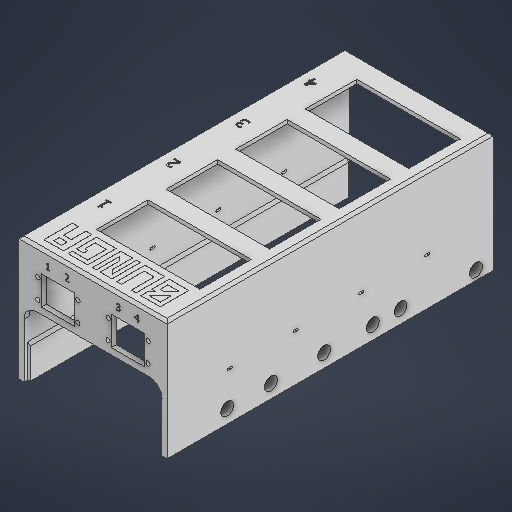
# Autodesk Inventor part: QuadSupply
Saved by Autodesk Inventor 2026 (Build 300175050, 175E)
## iProperties
Created: 2025-08-17
Part Number: QuadSupply
Material: Generic
Document SubType Name: Modeling
Designer: user
Density: 1 g/cm^3
Appearance: Default
Author: user
## iProperties of the stored document QuadSupply_3DPrint.ipt
Created: 2025-08-17
Part Number: QuadSupply_3DPrint
Material: Generic
Document SubType Name: Modeling
Designer: user
Density: 1 g/cm^3
Appearance: Default
Author: user
Autodesk Inventor part; units mm, degrees
ref_plane "YZ Plane" through (0, 0, 0) normal (1, 0, 0) x (0, 1, 0)
ref_plane "XZ Plane" through (0, 0, 0) normal (0, 1, 0) x (-1, 0, 0)
ref_plane "XY Plane" through (0, 0, 0) normal (0, 0, 1) x (1, 0, 0)
sketch "Sketch1" plane through (0, 0, 0) normal (0, 1, 0) x (-1, 0, 0)
  line L0 (54.5, -128.75) -> (-54.5, -128.75) construction
  line L1 (-54.5, -128.75) -> (-54.5, 128.75) construction
  line L2 (-54.5, 128.75) -> (54.5, 128.75) construction
  line L3 (54.5, 128.75) -> (54.5, -128.75) construction
  line L4 (58.5, -128.75) -> (-58.5, -128.75)
  line L5 (-58.5, -128.75) -> (-58.5, 128.75)
  line L6 (-58.5, 128.75) -> (58.5, 128.75)
  line L7 (58.5, 128.75) -> (58.5, -128.75)
  line L8 (32.1, -111.75) -> (-49.5, -111.75)
  line L9 (-49.5, -111.75) -> (-49.5, -71.15)
  line L10 (-49.5, -71.15) -> (32.1, -71.15)
  line L11 (32.1, -71.15) -> (32.1, -111.75)
  point P0 (0, 0)
  point P1 (-54.5, 0)
  point P2 (0, -128.75)
  point P3 (0, -128.75)
  point P4 (-58.5, 0)
  dimension "d0" = 109
  dimension "d1" = 257.5
  dimension "d3" = 4
  dimension "d4" = 40.6
  dimension "d5" = 81.6
  dimension "d6" = 17
  dimension "d56" = 5
  constraints: 24 end point, 6 parallel, 4 midpoint, 3 horizontal, 3 perpendicular, 2 horizontal alignment, 2 vertical alignment, 1 collinear
  measures "d0" distance of L0.start L0.end
  measures "d1" distance of L2.end L0.start
  measures "d3" distance between parallel lines of L3 L7
  measures "d4" distance of L10.end L8.start
  measures "d5" distance of L8.start L8.end
  measures "d6" distance between parallel lines of L4 L8
  measures "d56" distance between parallel lines of L1 L9
extrude "Extrusion1" add sketch "Sketch1" against normal blind 3 contours L4 L5 L6 L7 | L8 L9 L10 L11
extrude "Extrusion2" cut sketch "Sketch1" against normal up to surface (3 mm away) contours L8 L9 L10 L11
pattern_linear "Rectangular Pattern1" count 4 spacing 55 along (0, 0, 1) of "Extrusion2"
sketch "Sketch2" plane through (0, -3, 0) normal (0, -1, 0) x (1, 0, 0)
  line L0 (-58.5, -128.75) -> (-58.5, 128.75) projected
  line L1 (58.5, -128.75) -> (-58.5, -128.75) projected
  line L2 (-58.5, 128.75) -> (-54.5, 128.75)
  line L3 (-54.5, 128.75) -> (-54.5, -128.75)
  line L4 (-54.5, -128.75) -> (-58.5, -128.75)
  line L5 (-58.5, -128.75) -> (-58.5, 128.75)
  point P0 (0, 0)
  dimension "d15" = 4
  constraints: 8 end point, 2 parallel, 1 horizontal, 1 perpendicular, 1 point on line
  measures "d15" distance between parallel lines of L0 L3
extrude "Extrusion3" add sketch "Sketch2" along normal blind 95
sketch "Sketch3" plane through (-54.5, -3, 128.75) normal (1, 0, 0) x (0, 0, -1)
  line L0 (3, -69) -> (254.5, -69)
  line L1 (254.5, -69) -> (254.5, -95)
  line L2 (254.5, -95) -> (3, -95)
  line L3 (3, -95) -> (3, -69)
  line L4 (257.5, -95) -> (0, -95) projected
  point P0 (128.75, 3)
  point P1 (128.75, -95)
  dimension "d18" = 251.5
  dimension "d19" = 26
  constraints: 8 end point, 2 midpoint, 2 parallel, 1 horizontal, 1 perpendicular
  measures "d18" distance of L0.start L0.end
  measures "d19" distance between parallel lines of L2 L0
extrude "Extrusion4" add sketch "Sketch3" along normal blind 2
sketch "Sketch5" plane through (0, -3, 0) normal (0, -1, 0) x (1, 0, 0)
  line L0 (54.5, 128.75) -> (58.5, 128.75)
  line L1 (58.5, 128.75) -> (58.5, -128.75)
  line L2 (58.5, -128.75) -> (54.5, -128.75)
  line L3 (54.5, -128.75) -> (54.5, 128.75)
  point P0 (0, 0)
  dimension "d24" = 4
  constraints: 8 end point, 2 coincident, 2 parallel, 1 horizontal, 1 perpendicular
  measures "d24" distance between parallel lines of L1 L3
extrude "Extrusion5" add sketch "Sketch5" along normal blind 91.1
sketch "Sketch6" plane through (54.5, -3, -128.75) normal (-1, 0, 0) x (0, 0, 1)
  line L0 (3, -72.8) -> (254.5, -72.8)
  line L1 (254.5, -72.8) -> (254.5, -91.1)
  line L2 (254.5, -91.1) -> (3, -91.1)
  line L3 (3, -91.1) -> (3, -72.8)
  line L4 (257.5, -91.1) -> (0, -91.1) projected
  point P0 (128.75, 3)
  point P1 (128.75, -91.1)
  dimension "d27" = 251.5
  dimension "d28" = 18.3
  constraints: 8 end point, 2 midpoint, 2 parallel, 1 horizontal, 1 perpendicular
  measures "d27" distance of L0.start L0.end
  measures "d28" distance between parallel lines of L0 L2
extrude "Extrusion6" add sketch "Sketch6" along normal blind 3
sketch "Sketch7" plane through (51.5, -3, -128.75) normal (-1, 0, 0) x (0, 0, 1)
  line L0 (3, -72.8) -> (3, -91.1) projected
  line L1 (3, -91.1) -> (254.5, -91.1) projected
  line L2 (254.5, -91.1) -> (254.5, -72.8) projected
  line L3 (254.5, -72.8) -> (3, -72.8) projected
  line L4 (3, -80.6) -> (254.5, -80.6) construction
  line L5 (257.5, 0) -> (257.5, -91.1) projected
  circle A0 centre (210, -80.6) radius 5
  circle A1 centre (175.5, -80.6) radius 5
  circle A2 centre (133.5, -80.6) radius 5
  circle A3 centre (95, -80.6) radius 5
  circle A4 centre (73, -80.6) radius 5
  circle A5 centre (13.5, -83.9) radius 5
  point P0 (128.75, 3)
  dimension "d31" = 10.5
  dimension "d34" = 47.5
  dimension "d35" = 82
  dimension "d37" = 124
  dimension "d39" = 162.5
  dimension "d41" = 184.5
  dimension "d42" = 10
  dimension "d43" = 244
  dimension "d44" = 7.2
  constraints: 7 point on line, 6 centre point, 5 equal radius, 2 end point, 1 horizontal
  measures "d31" distance between parallel lines of L1 L4
  measures "d34" distance from line of L5 A0.centre
  measures "d35" distance from line of L5 A1.centre
  measures "d37" distance from line of L5 A2.centre
  measures "d39" distance from line of L5 A3.centre
  measures "d41" distance from line of L5 A4.centre
  measures "d42" diameter of A5
  measures "d43" distance from line of L5 A5.centre
  measures "d44" distance from line of L1 A5.centre
extrude "Extrusion7" cut sketch "Sketch7" against normal up to surface (7 mm away) contours A0 | A1 | A2 | A3 | A4 | A5
sketch "Sketch8" plane through (-58.5, 0, -128.75) normal (-1, 0, 0) x (0, 0, 1)
  line L0 (0, -58) -> (257.5, -58) construction
  line L1 (0, 0) -> (0, -98) projected
  line L2 (257.5, 0) -> (257.5, -98) projected
  line L3 (257.5, -98) -> (0, -98) projected
  line L4 (50.85, -57.15) -> (53.15, -57.15) construction
  line L5 (50.85, -58) -> (53.15, -58)
  line L6 (53.15, -56.3) -> (50.85, -56.3)
  arc A0 (50.85, -56.3) -> (50.85, -58) centre (50.85, -57.15) ccw
  arc A1 (53.15, -58) -> (53.15, -56.3) centre (53.15, -57.15) ccw
  point P0 (128.75, 0)
  point P1 (52, -57.15)
  point P2 (54, -57.15)
  point P3 (50, -57.15)
  point P4 (52, -58)
  dimension "d47" = 40
  dimension "d48" = 1.7
  dimension "d49" = 4
  dimension "d50" = 52
  constraints: 10 end point, 6 point on circle, 4 tangent, 3 point on line, 2 centre point, 2 horizontal, 2 midpoint, 1 parallel
  measures "d47" distance between parallel lines of L3 L0
  measures "d48" distance between parallel lines of L5 L6
  measures "d49" distance of point (54, -57.15) point (50, -57.15)
  measures "d50" distance from line of L1 point (52, -57.15)
extrude "Extrusion8" cut sketch "Sketch8" against normal up to surface (117 mm away)
pattern_linear "Rectangular Pattern2" count 4 spacing 52 along (0, 0, 1) of "Extrusion8"
sketch "Sketch9" plane through (-58.5, 0, 128.75) normal (0, 0, 1) x (1, 0, 0)
  line L0 (0, 0) -> (117, 0) projected
  line L1 (0, 0) -> (0, -98) projected
  line L2 (117, 0) -> (0, 0)
  line L3 (0, 0) -> (0, -45)
  line L4 (0, -45) -> (117, -45)
  line L5 (117, -45) -> (117, 0)
  point P0 (58.5, 0)
  dimension "d57" = 45
  constraints: 8 end point, 2 parallel, 1 horizontal, 1 perpendicular, 1 point on line
  measures "d57" distance between parallel lines of L0 L4
extrude "Extrusion9" add sketch "Sketch9" against normal blind 4
sketch "Sketch10" plane through (-58.5, 0, 128.75) normal (0, 0, 1) x (1, 0, 0)
  line L0 (15, -20.85) -> (46.6, -20.85) construction
  line L1 (46.6, -20.85) -> (46.6, -36.35) construction
  line L2 (46.6, -36.35) -> (15, -36.35) construction
  line L3 (15, -36.35) -> (15, -20.85) construction
  circle A0 centre (15, -20.85) radius 1.65
  circle A1 centre (46.6, -20.85) radius 1.65
  circle A2 centre (15, -36.35) radius 1.65
  circle A3 centre (46.6, -36.35) radius 1.65
  line L4 (17.6, -17.2) -> (44, -17.2)
  line L5 (44, -17.2) -> (44, -40)
  line L6 (44, -40) -> (17.6, -40)
  line L7 (17.6, -40) -> (17.6, -17.2)
  line L8 (4, -45) -> (113, -45) projected
  line L9 (0, 0) -> (0, -98) projected
  line L10 (70.4, -20.85) -> (102, -20.85) construction
  line L11 (102, -20.85) -> (102, -36.35) construction
  line L12 (102, -36.35) -> (70.4, -36.35) construction
  line L13 (70.4, -36.35) -> (70.4, -20.85) construction
  circle A4 centre (70.4, -20.85) radius 1.65
  circle A5 centre (102, -20.85) radius 1.65
  circle A6 centre (70.4, -36.35) radius 1.65
  circle A7 centre (102, -36.35) radius 1.65
  line L14 (73, -17.2) -> (99.4, -17.2)
  line L15 (99.4, -17.2) -> (99.4, -40)
  line L16 (99.4, -40) -> (73, -40)
  line L17 (73, -40) -> (73, -17.2)
  line L18 (117, 0) -> (117, -94.1) projected
  point P0 (58.5, 0)
  point P1 (30.8, -20.85)
  point P2 (30.8, -17.2)
  point P3 (44, -28.6)
  point P4 (46.6, -28.6)
  point P5 (86.2, -20.85)
  point P6 (86.2, -17.2)
  point P7 (99.4, -28.6)
  point P8 (102, -28.6)
  dimension "d60" = 31.6
  dimension "d61" = 15.5
  dimension "d62" = 3.3
  dimension "d63" = 26.4
  dimension "d64" = 22.8
  dimension "d65" = 5
  dimension "d66" = 15
  dimension "d67" = 31.6
  dimension "d68" = 15.5
  dimension "d69" = 3.3
  dimension "d70" = 26.4
  dimension "d71" = 22.8
  dimension "d72" = 15
  dimension "d73" = 5
  constraints: 32 end point, 8 centre point, 8 coincident, 8 midpoint, 8 parallel, 6 equal radius, 4 horizontal, 4 perpendicular, 2 horizontal alignment, 2 vertical alignment
  measures "d60" distance of L0.start L0.end
  measures "d61" distance of L2.end L0.start
  measures "d62" diameter of A0
  measures "d63" distance of L4.start L4.end
  measures "d64" distance of L4.end L5.end
  measures "d65" distance between parallel lines of L8 L6
  measures "d66" distance between parallel lines of L9 L3
  measures "d67" distance of L13.end L11.start
  measures "d68" distance of L13.start L13.end
  measures "d69" diameter of A4
  measures "d70" distance of L14.start L14.end
  measures "d71" distance of L14.end L15.end
  measures "d72" distance between parallel lines of L18 L11
  measures "d73" distance between parallel lines of L8 L16
extrude "Extrusion10" cut sketch "Sketch10" against normal up to surface (4 mm away)
sketch "Sketch11" plane through (-58.5, 0, 128.75) normal (0, 0, 1) x (1, 0, 0)
  line L0 (20.9646, -7.3633) -> (24.7195, -7.3633) construction
  line L1 (24.7195, -7.3633) -> (24.7195, -12.4045) construction
  line L2 (24.7195, -12.4045) -> (20.9646, -12.4045) construction
  line L3 (20.9646, -12.4045) -> (20.9646, -7.3633) construction
  line L4 (36.1808, -7.3633) -> (39.9357, -7.3633) construction
  line L5 (39.9357, -7.3633) -> (39.9357, -12.4045) construction
  line L6 (39.9357, -12.4045) -> (36.1808, -12.4045) construction
  line L7 (36.1808, -12.4045) -> (36.1808, -7.3633) construction
  line L8 (76.6169, -7.3633) -> (80.3717, -7.3633) construction
  line L9 (80.3717, -7.3633) -> (80.3717, -12.4045) construction
  line L10 (80.3717, -12.4045) -> (76.6169, -12.4045) construction
  line L11 (76.6169, -12.4045) -> (76.6169, -7.3633) construction
  line L12 (91.1541, -7.3633) -> (94.9089, -7.3633) construction
  line L13 (94.9089, -7.3633) -> (94.9089, -12.4045) construction
  line L14 (94.9089, -12.4045) -> (91.1541, -12.4045) construction
  line L15 (91.1541, -12.4045) -> (91.1541, -7.3633) construction
  line L16 (24.164, -12.3833) -> (21.7229, -12.3833)
  line L17 (21.7229, -12.3833) -> (21.7229, -11.8724)
  line L18 (21.7229, -11.8724) -> (22.6312, -11.8724)
  line L19 (22.6312, -11.8724) -> (22.6312, -8.519)
  line L20 (22.6312, -8.519) -> (21.7229, -8.519)
  line L21 (21.7229, -8.519) -> (21.7229, -8.0608)
  spline S0 degree 2 poles (21.7229, -8.0608) (22.2379, -8.0608) (22.7245, -7.7688) (22.7569, -7.3633) knots 0 0 0 1 2 2 2
  line L22 (22.7569, -7.3633) -> (23.2759, -7.3633)
  line L23 (23.2759, -7.3633) -> (23.2759, -11.8724)
  line L24 (23.2759, -11.8724) -> (24.164, -11.8724)
  line L25 (24.164, -11.8724) -> (24.164, -12.3833)
  line L26 (39.6315, -12.4725) -> (36.5457, -12.4725)
  line L27 (36.5457, -12.4725) -> (36.5457, -11.7629)
  spline S1 degree 2 poles (36.5457, -11.7629) (36.8782, -11.4507) (37.4703, -10.8708) (37.7541, -10.5586) knots 0 0 0 1 2 2 2
  spline S2 degree 2 poles (37.7541, -10.5586) (38.3258, -9.9301) (38.7435, -9.1759) (38.7435, -8.7744) knots 0 0 0 1 2 2 2
  spline S3 degree 2 poles (38.7435, -8.7744) (38.7435, -8.5636) (38.6137, -8.2473) (38.4962, -8.1459) knots 0 0 0 1 2 2 2
  spline S4 degree 2 poles (38.4962, -8.1459) (38.3786, -8.0445) (38.0704, -7.9432) (37.8839, -7.9432) knots 0 0 0 1 2 2 2
  spline S5 degree 2 poles (37.8839, -7.9432) (37.7054, -7.9432) (37.3405, -8.0324) (37.1742, -8.1013) knots 0 0 0 1 2 2 2
  spline S6 degree 2 poles (37.1742, -8.1013) (37.0323, -8.1581) (36.7688, -8.3203) (36.6877, -8.377) knots 0 0 0 1 2 2 2
  line L28 (36.6877, -8.377) -> (36.6512, -8.377)
  line L29 (36.6512, -8.377) -> (36.6512, -7.6634)
  spline S7 degree 2 poles (36.6512, -7.6634) (36.858, -7.562) (37.6, -7.3633) (37.9325, -7.3633) knots 0 0 0 1 2 2 2
  spline S8 degree 2 poles (37.9325, -7.3633) (38.634, -7.3633) (39.4247, -8.1054) (39.4247, -8.7379) knots 0 0 0 1 2 2 2
  spline S9 degree 2 poles (39.4247, -8.7379) (39.4247, -9.0339) (39.2869, -9.5286) (39.1652, -9.7395) knots 0 0 0 1 2 2 2
  spline S10 degree 2 poles (39.1652, -9.7395) (39.0436, -9.9585) (38.6908, -10.3883) (38.4962, -10.5951) knots 0 0 0 1 2 2 2
  spline S11 degree 2 poles (38.4962, -10.5951) (38.1799, -10.9398) (37.4054, -11.6778) (37.1742, -11.8927) knots 0 0 0 1 2 2 2
  line L30 (37.1742, -11.8927) -> (39.6315, -11.8927)
  line L31 (39.6315, -11.8927) -> (39.6315, -12.4725)
  spline S12 degree 2 poles (78.3321, -7.9432) (78.1496, -7.9432) (77.7887, -8.0324) (77.6144, -8.1013) knots 0 0 0 1 2 2 2
  spline S13 degree 2 poles (77.6144, -8.1013) (77.4522, -8.1702) (77.2129, -8.3162) (77.1197, -8.3811) knots 0 0 0 1 2 2 2
  line L32 (77.1197, -8.3811) -> (77.0791, -8.3811)
  line L33 (77.0791, -8.3811) -> (77.0791, -7.6715)
  spline S14 degree 2 poles (77.0791, -7.6715) (77.2981, -7.5539) (78.0483, -7.3633) (78.3848, -7.3633) knots 0 0 0 1 2 2 2
  spline S15 degree 2 poles (78.3848, -7.3633) (78.7254, -7.3633) (79.2323, -7.5012) (79.4391, -7.6472) knots 0 0 0 1 2 2 2
  spline S16 degree 2 poles (79.4391, -7.6472) (79.6581, -7.8053) (79.8852, -8.2635) (79.8852, -8.5717) knots 0 0 0 1 2 2 2
  spline S17 degree 2 poles (79.8852, -8.5717) (79.8852, -8.9853) (79.3418, -9.6097) (78.9606, -9.6908) knots 0 0 0 1 2 2 2
  line L34 (78.9606, -9.6908) -> (78.9606, -9.7395)
  spline S18 degree 2 poles (78.9606, -9.7395) (79.1188, -9.7719) (79.4797, -9.9179) (79.6337, -10.0639) knots 0 0 0 1 2 2 2
  spline S19 degree 2 poles (79.6337, -10.0639) (79.7878, -10.2058) (79.9825, -10.66) (79.9825, -10.9884) knots 0 0 0 1 2 2 2
  spline S20 degree 2 poles (79.9825, -10.9884) (79.9825, -11.325) (79.7513, -11.8967) (79.5405, -12.1157) knots 0 0 0 1 2 2 2
  spline S21 degree 2 poles (79.5405, -12.1157) (79.3215, -12.3428) (78.7011, -12.578) (78.3078, -12.578) knots 0 0 0 1 2 2 2
  spline S22 degree 2 poles (78.3078, -12.578) (77.9307, -12.578) (77.1927, -12.3955) (76.9413, -12.2698) knots 0 0 0 1 2 2 2
  line L35 (76.9413, -12.2698) -> (76.9413, -11.5602)
  line L36 (76.9413, -11.5602) -> (76.9899, -11.5602)
  spline S23 degree 2 poles (76.9899, -11.5602) (77.2008, -11.7143) (77.9145, -11.9981) (78.2672, -11.9981) knots 0 0 0 1 2 2 2
  spline S24 degree 2 poles (78.2672, -11.9981) (78.474, -11.9981) (78.8876, -11.8683) (79.0255, -11.7183) knots 0 0 0 1 2 2 2
  spline S25 degree 2 poles (79.0255, -11.7183) (79.1593, -11.5683) (79.3012, -11.2114) (79.3012, -10.9398) knots 0 0 0 1 2 2 2
  spline S26 degree 2 poles (79.3012, -10.9398) (79.3012, -10.6681) (79.1431, -10.3153) (79.0012, -10.2139) knots 0 0 0 1 2 2 2
  spline S27 degree 2 poles (79.0012, -10.2139) (78.8593, -10.1126) (78.474, -10.0355) (78.247, -10.0355) knots 0 0 0 1 2 2 2
  line L37 (78.247, -10.0355) -> (77.9631, -10.0355)
  line L38 (77.9631, -10.0355) -> (77.9631, -9.48)
  line L39 (77.9631, -9.48) -> (78.1861, -9.48)
  spline S28 degree 2 poles (78.1861, -9.48) (78.6362, -9.48) (79.2039, -9.0502) (79.2039, -8.6406) knots 0 0 0 1 2 2 2
  spline S29 degree 2 poles (79.2039, -8.6406) (79.2039, -8.45) (79.0579, -8.1783) (78.9404, -8.0972) knots 0 0 0 1 2 2 2
  spline S30 degree 2 poles (78.9404, -8.0972) (78.8146, -8.0121) (78.5065, -7.9432) (78.3321, -7.9432) knots 0 0 0 1 2 2 2
  line L40 (94.7386, -10.6478) -> (94.1425, -10.6478)
  line L41 (94.1425, -10.6478) -> (94.1425, -12.3671)
  line L42 (94.1425, -12.3671) -> (93.4978, -12.3671)
  line L43 (93.4978, -12.3671) -> (93.4978, -10.6478)
  line L44 (93.4978, -10.6478) -> (91.2879, -10.6478)
  line L45 (91.2879, -10.6478) -> (91.2879, -9.9422)
  line L46 (91.2879, -9.9422) -> (93.5262, -7.3633)
  line L47 (93.5262, -7.3633) -> (94.1425, -7.3633)
  line L48 (94.1425, -7.3633) -> (94.1425, -10.1085)
  line L49 (94.1425, -10.1085) -> (94.7386, -10.1085)
  line L50 (94.7386, -10.1085) -> (94.7386, -10.6478)
  line L51 (93.4978, -10.1085) -> (93.4978, -8.154)
  line L52 (93.4978, -8.154) -> (91.815, -10.1085)
  line L53 (91.815, -10.1085) -> (93.4978, -10.1085)
  point P0 (58.5, 0)
  point P1 (24.7195, -9.8839)
  point P2 (36.1808, -9.8839)
  point P3 (76.6169, -9.8839)
  point P4 (91.1541, -9.8839)
  dimension "d0" = 109
  dimension "d1" = 257.5
  dimension "d3" = 4
  dimension "d4" = 40.6
  dimension "d5" = 81.6
  dimension "d6" = 17
  dimension "d56" = 5
  constraints: 4 midpoint, 3 collinear, 3 horizontal alignment, 8 other
extrude "Extrusion11" cut sketch "Sketch11" against normal blind 0.5
sketch "Sketch12" plane through (0, 0, 0) normal (0, 1, 0) x (1, 0, 0)
  line L0 (-43.6132, -77.5449) -> (-49.3868, -77.5449) construction
  line L1 (-49.3868, -77.5449) -> (-49.3868, -69.5551) construction
  line L2 (-49.3868, -69.5551) -> (-43.6132, -69.5551) construction
  line L3 (-43.6132, -69.5551) -> (-43.6132, -77.5449) construction
  line L4 (-44.2509, -22.5844) -> (-48.7491, -22.5844) construction
  line L5 (-48.7491, -22.5844) -> (-48.7491, -14.5156) construction
  line L6 (-48.7491, -14.5156) -> (-44.2509, -14.5156) construction
  line L7 (-44.2509, -14.5156) -> (-44.2509, -22.5844) construction
  line L8 (-44.2764, 32.2784) -> (-48.7236, 32.2784) construction
  line L9 (-48.7236, 32.2784) -> (-48.7236, 40.6216) construction
  line L10 (-48.7236, 40.6216) -> (-44.2764, 40.6216) construction
  line L11 (-44.2764, 40.6216) -> (-44.2764, 32.2784) construction
  line L12 (-44.7542, 87.4582) -> (-48.2458, 87.4582) construction
  line L13 (-48.2458, 87.4582) -> (-48.2458, 95.4418) construction
  line L14 (-48.2458, 95.4418) -> (-44.7542, 95.4418) construction
  line L15 (-44.7542, 95.4418) -> (-44.7542, 87.4582) construction
  line L16 (-32.1, -93.85) -> (-32.1, -53.25) projected
  line L17 (-32.1, -38.85) -> (-32.1, 1.75) projected
  line L18 (-32.1, 16.15) -> (-32.1, 56.75) projected
  line L19 (-32.1, 71.15) -> (-32.1, 111.75) projected
  line L20 (-58.5, 128.75) -> (-58.5, -128.75) projected
  line L21 (-48.7289, -69.5179) -> (-44.8257, -69.5179)
  line L22 (-44.8257, -69.5179) -> (-44.8257, -70.3349)
  line L23 (-44.8257, -70.3349) -> (-46.278, -70.3349)
  line L24 (-46.278, -70.3349) -> (-46.278, -75.697)
  line L25 (-46.278, -75.697) -> (-44.8257, -75.697)
  line L26 (-44.8257, -75.697) -> (-44.8257, -76.4296)
  spline S0 degree 2 poles (-44.8257, -76.4296) (-45.6491, -76.4296) (-46.4271, -76.8965) (-46.479, -77.5449) knots 0 0 0 1 2 2 2
  line L27 (-46.479, -77.5449) -> (-47.3089, -77.5449)
  line L28 (-47.3089, -77.5449) -> (-47.3089, -70.3349)
  line L29 (-47.3089, -70.3349) -> (-48.7289, -70.3349)
  line L30 (-48.7289, -70.3349) -> (-48.7289, -69.5179)
  line L31 (-49.7686, -14.4148) -> (-44.8344, -14.4148)
  line L32 (-44.8344, -14.4148) -> (-44.8344, -15.5495)
  spline S1 degree 2 poles (-44.8344, -15.5495) (-45.3661, -16.0487) (-46.3127, -16.9759) (-46.7666, -17.4751) knots 0 0 0 1 2 2 2
  spline S2 degree 2 poles (-46.7666, -17.4751) (-47.6808, -18.4801) (-48.3486, -19.6861) (-48.3486, -20.328) knots 0 0 0 1 2 2 2
  spline S3 degree 2 poles (-48.3486, -20.328) (-48.3486, -20.6652) (-48.1412, -21.1709) (-47.9531, -21.333) knots 0 0 0 1 2 2 2
  spline S4 degree 2 poles (-47.9531, -21.333) (-47.7651, -21.4951) (-47.2723, -21.6572) (-46.9741, -21.6572) knots 0 0 0 1 2 2 2
  spline S5 degree 2 poles (-46.9741, -21.6572) (-46.6888, -21.6572) (-46.1053, -21.5145) (-45.8394, -21.4043) knots 0 0 0 1 2 2 2
  spline S6 degree 2 poles (-45.8394, -21.4043) (-45.6125, -21.3136) (-45.191, -21.0542) (-45.0614, -20.9634) knots 0 0 0 1 2 2 2
  line L33 (-45.0614, -20.9634) -> (-45.003, -20.9634)
  line L34 (-45.003, -20.9634) -> (-45.003, -22.1046)
  spline S7 degree 2 poles (-45.003, -22.1046) (-45.3337, -22.2667) (-46.5202, -22.5844) (-47.0519, -22.5844) knots 0 0 0 1 2 2 2
  spline S8 degree 2 poles (-47.0519, -22.5844) (-48.1736, -22.5844) (-49.4379, -21.3978) (-49.4379, -20.3864) knots 0 0 0 1 2 2 2
  spline S9 degree 2 poles (-49.4379, -20.3864) (-49.4379, -19.9131) (-49.2175, -19.122) (-49.023, -18.7849) knots 0 0 0 1 2 2 2
  spline S10 degree 2 poles (-49.023, -18.7849) (-48.8284, -18.4347) (-48.2644, -17.7475) (-47.9531, -17.4168) knots 0 0 0 1 2 2 2
  spline S11 degree 2 poles (-47.9531, -17.4168) (-47.4474, -16.8657) (-46.209, -15.6856) (-45.8394, -15.342) knots 0 0 0 1 2 2 2
  line L35 (-45.8394, -15.342) -> (-49.7686, -15.342)
  line L36 (-49.7686, -15.342) -> (-49.7686, -14.4148)
  spline S12 degree 2 poles (-47.0191, 33.2055) (-46.7273, 33.2055) (-46.1503, 33.3482) (-45.8715, 33.4584) knots 0 0 0 1 2 2 2
  spline S13 degree 2 poles (-45.8715, 33.4584) (-45.6121, 33.5686) (-45.2296, 33.802) (-45.0804, 33.9058) knots 0 0 0 1 2 2 2
  line L37 (-45.0804, 33.9058) -> (-45.0156, 33.9058)
  line L38 (-45.0156, 33.9058) -> (-45.0156, 32.7711)
  spline S14 degree 2 poles (-45.0156, 32.7711) (-45.3657, 32.5831) (-46.5652, 32.2784) (-47.1034, 32.2784) knots 0 0 0 1 2 2 2
  spline S15 degree 2 poles (-47.1034, 32.2784) (-47.648, 32.2784) (-48.4585, 32.4988) (-48.7892, 32.7322) knots 0 0 0 1 2 2 2
  spline S16 degree 2 poles (-48.7892, 32.7322) (-49.1393, 32.9851) (-49.5024, 33.7178) (-49.5024, 34.2105) knots 0 0 0 1 2 2 2
  spline S17 degree 2 poles (-49.5024, 34.2105) (-49.5024, 34.8719) (-48.6336, 35.8704) (-48.0241, 36.0001) knots 0 0 0 1 2 2 2
  line L39 (-48.0241, 36.0001) -> (-48.0241, 36.0779)
  spline S18 degree 2 poles (-48.0241, 36.0779) (-48.2769, 36.1297) (-48.854, 36.3631) (-49.1004, 36.5966) knots 0 0 0 1 2 2 2
  spline S19 degree 2 poles (-49.1004, 36.5966) (-49.3468, 36.8235) (-49.658, 37.5497) (-49.658, 38.0749) knots 0 0 0 1 2 2 2
  spline S20 degree 2 poles (-49.658, 38.0749) (-49.658, 38.613) (-49.2884, 39.5272) (-48.9513, 39.8774) knots 0 0 0 1 2 2 2
  spline S21 degree 2 poles (-48.9513, 39.8774) (-48.6011, 40.2405) (-47.6091, 40.6165) (-46.9802, 40.6165) knots 0 0 0 1 2 2 2
  spline S22 degree 2 poles (-46.9802, 40.6165) (-46.3772, 40.6165) (-45.1971, 40.3247) (-44.7951, 40.1237) knots 0 0 0 1 2 2 2
  line L40 (-44.7951, 40.1237) -> (-44.7951, 38.9891)
  line L41 (-44.7951, 38.9891) -> (-44.873, 38.9891)
  spline S23 degree 2 poles (-44.873, 38.9891) (-45.2101, 39.2355) (-46.3513, 39.6893) (-46.9153, 39.6893) knots 0 0 0 1 2 2 2
  spline S24 degree 2 poles (-46.9153, 39.6893) (-47.246, 39.6893) (-47.9074, 39.4819) (-48.1278, 39.242) knots 0 0 0 1 2 2 2
  spline S25 degree 2 poles (-48.1278, 39.242) (-48.3418, 39.0021) (-48.5687, 38.4315) (-48.5687, 37.9971) knots 0 0 0 1 2 2 2
  spline S26 degree 2 poles (-48.5687, 37.9971) (-48.5687, 37.5626) (-48.3158, 36.9986) (-48.0889, 36.8365) knots 0 0 0 1 2 2 2
  spline S27 degree 2 poles (-48.0889, 36.8365) (-47.862, 36.6744) (-47.246, 36.5512) (-46.8829, 36.5512) knots 0 0 0 1 2 2 2
  line L42 (-46.8829, 36.5512) -> (-46.4291, 36.5512)
  line L43 (-46.4291, 36.5512) -> (-46.4291, 35.6629)
  line L44 (-46.4291, 35.6629) -> (-46.7857, 35.6629)
  spline S28 degree 2 poles (-46.7857, 35.6629) (-47.5054, 35.6629) (-48.4131, 34.9756) (-48.4131, 34.3208) knots 0 0 0 1 2 2 2
  spline S29 degree 2 poles (-48.4131, 34.3208) (-48.4131, 34.016) (-48.1797, 33.5816) (-47.9917, 33.4519) knots 0 0 0 1 2 2 2
  spline S30 degree 2 poles (-47.9917, 33.4519) (-47.7907, 33.3158) (-47.2979, 33.2055) (-47.0191, 33.2055) knots 0 0 0 1 2 2 2
  line L45 (-50.4859, 92.7101) -> (-49.5328, 92.7101)
  line L46 (-49.5328, 92.7101) -> (-49.5328, 95.4592)
  line L47 (-49.5328, 95.4592) -> (-48.5019, 95.4592)
  line L48 (-48.5019, 95.4592) -> (-48.5019, 92.7101)
  line L49 (-48.5019, 92.7101) -> (-44.9682, 92.7101)
  line L50 (-44.9682, 92.7101) -> (-44.9682, 91.5819)
  line L51 (-44.9682, 91.5819) -> (-48.5473, 87.4582)
  line L52 (-48.5473, 87.4582) -> (-49.5328, 87.4582)
  line L53 (-49.5328, 87.4582) -> (-49.5328, 91.8478)
  line L54 (-49.5328, 91.8478) -> (-50.4859, 91.8478)
  line L55 (-50.4859, 91.8478) -> (-50.4859, 92.7101)
  line L56 (-48.5019, 91.8478) -> (-48.5019, 88.7226)
  line L57 (-48.5019, 88.7226) -> (-45.8111, 91.8478)
  line L58 (-45.8111, 91.8478) -> (-48.5019, 91.8478)
  point P0 (0, 0)
  point P1 (-32.1, -73.55)
  point P2 (-43.6132, -73.55)
  point P3 (-32.1, -18.55)
  point P4 (-44.2509, -18.55)
  point P5 (-32.1, 36.45)
  point P6 (-44.2764, 36.45)
  point P7 (-32.1, 91.45)
  point P8 (-44.7542, 91.45)
  point P9 (-46.5, -69.5551)
  point P10 (-46.5, -14.5156)
  point P11 (-46.5, 40.6216)
  point P12 (-46.5, 95.4418)
  dimension "d0" = 109
  dimension "d1" = 257.5
  dimension "d3" = 4
  dimension "d4" = 40.6
  dimension "d5" = 81.6
  dimension "d6" = 17
  dimension "d56" = 5
  dimension "d178" = 12
  constraints: 12 midpoint, 4 horizontal alignment, 3 vertical alignment, 8 other
  measures "d178" distance from line of L20 point (-46.5, -69.555)
extrude "Extrusion12" cut sketch "Sketch12" against normal blind 0.5
chamfer "Chamfer1" distance 2 angle 45 7 edges at (54.5, -3, -2) (-54.5, -3, -2) (-58.5, 0, 0) (58.5, 0, 0) (0, 0, 128.75) (0, 0, -128.75) (0, -3, 124.75)
chamfer "Chamfer2" distance 3 angle 45 1 edges at (51.5, -75.8, 0)
chamfer "Chamfer3" distance 2 angle 45 1 edges at (-52.5, -72, 0)
fillet "Fillet1" radius 10 2 edges at (-54.5, -45, 126.75) (54.5, -45, 126.75)
sketch "Sketch13" plane through (0, 0, 0) normal (0, 1, 0) x (1, 0, 0)
  line L0 (12.43, -113.919) -> (-12.43, -113.919) construction
  line L1 (-12.43, -113.919) -> (-12.43, -106.681) construction
  line L2 (-12.43, -106.681) -> (12.43, -106.681) construction
  line L3 (12.43, -106.681) -> (12.43, -113.919) construction
  line L4 (49.5, -93.85) -> (-32.1, -93.85) construction
  line L5 (11.44, -121.52) -> (11.44, -99.08)
  line L6 (15.18, -121.52) -> (11.44, -121.52)
  line L7 (15.18, -103.48) -> (15.18, -121.52)
  line L8 (23.1, -103.48) -> (15.18, -103.48)
  line L9 (26.84, -99.08) -> (26.84, -121.52)
  line L10 (26.84, -121.52) -> (23.1, -121.52)
  line L11 (23.1, -121.52) -> (23.1, -103.48)
  line L12 (11.44, -99.08) -> (26.84, -99.08)
  line L13 (7.7, -99.08) -> (7.7, -121.52) construction
  line L14 (26.84, -121.52) -> (11.44, -121.52) construction
  line L15 (11.44, -99.08) -> (26.84, -99.08) construction
  line L16 (11.44, -121.52) -> (11.44, -99.08) construction
  line L17 (33.88, -109.6501) -> (33.88, -103.48)
  line L18 (30.58, -99.08) -> (30.58, -112.9501)
  line L19 (26.84, -99.08) -> (26.84, -121.52) construction
  line L20 (30.58, -121.52) -> (30.58, -99.08) construction
  line L21 (30.58, -99.08) -> (45.98, -99.08) construction
  line L22 (45.98, -99.08) -> (45.98, -121.52) construction
  line L23 (45.98, -121.52) -> (30.58, -121.52) construction
  line L24 (41.4706, -110.0527) -> (33.88, -117.6433)
  line L25 (33.88, -103.48) -> (42.68, -103.48)
  line L26 (42.68, -114.1364) -> (36.599, -114.1364) construction
  line L27 (33.88, -118.22) -> (42.68, -118.22)
  line L28 (45.98, -99.08) -> (30.58, -99.08)
  line L29 (30.58, -121.52) -> (45.98, -121.52)
  line L30 (45.98, -121.52) -> (45.98, -99.08)
  line L31 (42.68, -118.22) -> (42.68, -110.0527)
  line L32 (42.68, -110.0527) -> (41.4706, -110.0527)
  line L33 (188.5027, -109.1759) -> (237.2968, -109.1759) construction
  line L34 (42.68, -103.48) -> (42.68, -104.1501)
  line L35 (42.68, -104.1501) -> (37.18, -109.6501)
  line L36 (42.68, -104.1501) -> (48.9524, -104.1501) construction
  line L37 (7.7, -99.08) -> (7.7, -121.52) construction
  line L38 (11.44, -99.08) -> (26.84, -99.08) construction
  line L39 (26.84, -99.08) -> (26.84, -121.52) construction
  line L40 (26.84, -121.52) -> (11.44, -121.52) construction
  line L41 (-26.84, -99.08) -> (-11.44, -99.08) construction
  line L42 (7.7, -121.52) -> (-7.7, -121.52) construction
  line L43 (-11.44, -121.52) -> (-26.84, -121.52) construction
  line L44 (-7.7, -121.52) -> (-7.7, -99.08) construction
  line L45 (-7.7, -121.52) -> (-7.7, -99.08) construction
  line L46 (-7.7, -99.08) -> (7.7, -99.08) construction
  line L47 (0, -121.52) -> (0, -99.08) construction
  line L48 (1.54, -115.14) -> (4.62, -118.22)
  line L49 (4.62, -118.22) -> (4.62, -99.08)
  line L50 (4.62, -99.08) -> (7.7, -99.08)
  line L51 (1.54, -99.08) -> (1.54, -115.14)
  line L52 (-7.7, -121.52) -> (-7.7, -99.08) construction
  line L53 (-1.54, -121.52) -> (-1.54, -106.56)
  line L54 (7.7, -99.08) -> (7.7, -121.52)
  line L55 (7.7, -121.52) -> (-1.54, -121.52)
  line L56 (-7.7, -99.08) -> (7.7, -99.08) construction
  line L57 (7.7, -121.52) -> (-7.7, -121.52) construction
  line L58 (7.7, -99.08) -> (7.7, -121.52) construction
  line L59 (11.44, -121.52) -> (11.44, -99.08) construction
  line L60 (-7.7, -99.08) -> (7.7, -99.08) construction
  line L61 (7.7, -121.52) -> (-7.7, -121.52) construction
  line L62 (-26.84, -118.22) -> (-26.84, -121.52)
  line L63 (-30.58, -99.08) -> (-35.2, -99.08)
  line L64 (-41.36, -118.44) -> (-35.2, -118.44)
  line L65 (-30.58, -121.52) -> (-45.98, -121.52) construction
  line L66 (-45.98, -121.52) -> (-45.98, -99.08) construction
  line L67 (-45.98, -99.08) -> (-30.58, -99.08) construction
  line L68 (-35.2, -99.08) -> (-35.2, -110.74)
  line L69 (-35.2, -118.44) -> (-35.2, -114.04)
  line L70 (-35.2, -110.74) -> (-41.36, -110.74)
  line L71 (-41.36, -110.74) -> (-41.36, -99.08)
  line L72 (-30.58, -121.52) -> (-30.58, -99.08)
  line L73 (-35.2, -114.04) -> (-41.36, -114.04)
  line L74 (-41.36, -99.08) -> (-45.98, -99.08)
  line L75 (-41.36, -114.04) -> (-41.36, -118.44)
  line L76 (-45.98, -121.52) -> (-30.58, -121.52)
  line L77 (-45.98, -99.08) -> (-45.98, -121.52)
  line L78 (-26.84, -114.92) -> (-21.12, -114.92)
  line L79 (-21.12, -114.92) -> (-21.12, -111.62)
  line L80 (-21.12, -111.62) -> (-23.54, -111.62)
  line L81 (-14.74, -118.22) -> (-26.84, -118.22)
  line L82 (-11.44, -121.52) -> (-26.84, -121.52) construction
  line L83 (-26.84, -121.52) -> (-11.44, -121.52)
  line L84 (-23.54, -111.62) -> (-23.54, -103.48)
  line L85 (-14.74, -103.48) -> (-14.74, -118.22)
  line L86 (-23.54, -103.48) -> (-14.74, -103.48)
  line L87 (-11.44, -99.08) -> (-11.44, -121.52) construction
  line L88 (-26.84, -99.08) -> (-11.44, -99.08) construction
  line L89 (-11.44, -99.08) -> (-26.84, -99.08)
  line L90 (-26.84, -99.08) -> (-26.84, -114.92)
  line L91 (-26.84, -121.52) -> (-26.84, -99.08) construction
  line L92 (-30.58, -99.08) -> (-30.58, -121.52) construction
  line L93 (-26.84, -121.52) -> (-26.84, -99.08) construction
  line L94 (30.58, -121.52) -> (30.58, -116.2501)
  line L95 (33.88, -117.6433) -> (33.88, -118.22)
  line L96 (30.58, -116.2501) -> (35.2469, -116.2501) construction
  line L97 (30.58, -116.2501) -> (33.88, -112.9501)
  line L98 (33.88, -112.9501) -> (30.58, -112.9501)
  line L99 (33.88, -112.9501) -> (37.18, -109.6501) construction
  line L100 (37.18, -109.6501) -> (33.88, -109.6501)
  line L101 (32.8329, -110.3) -> (30.58, -110.3) construction
  line L102 (32.8329, -110.3) -> (30.58, -110.3)
  line L103 (-11.44, -99.08) -> (-11.44, -121.52) construction
  line L104 (-11.44, -121.52) -> (-11.44, -99.08)
  line L105 (-7.7, -121.52) -> (-7.7, -99.08)
  line L106 (-7.7, -99.08) -> (1.54, -99.08)
  line L107 (-4.62, -121.52) -> (-7.7, -121.52)
  line L108 (-4.62, -103.48) -> (-4.62, -121.52)
  line L109 (-1.54, -106.56) -> (-4.62, -103.48)
  point P0 (0, 0)
  point P1 (56.5, -126.75)
  point P2 (-56.5, -126.75)
  point P3 (0, -110.3)
  point P4 (0, -113.919)
  point P5 (-12.43, -110.3)
  point P6 (0, -110.3)
  point P7 (11.44, -110.3)
  point P8 (19.14, -121.52)
  point P9 (19.14, -121.52)
  point P10 (19.14, -110.3)
  point P11 (38.28, -121.52)
  point P12 (38.28, -110.3)
  point P13 (11.44, -110.3)
  point P14 (19.14, -110.3)
  point P15 (-19.14, -121.52)
  point P16 (-7.7, -110.3)
  point P17 (-7.7, -110.3)
  point P18 (-8.8, -110.3)
  point P19 (-19.14, -110.3)
  point P20 (0, -110.3)
  point P21 (-7.7, -110.3)
  point P22 (0, -110.3)
  point P23 (0, -121.52)
  point P24 (-19.14, -121.52)
  point P25 (-26.84, -110.3)
  point P26 (-38.28, -121.52)
  point P27 (-38.28, -110.3)
  point P28 (-45.98, -110.3)
  point P29 (-26.84, -110.3)
  point P30 (-19.14, -110.3)
  point P31 (28.27, -114.8629)
  point P32 (0, -110.3)
  point P33 (0, -110.3)
  dimension "d137" = 15.4
  dimension "d138" = 22.44
  dimension "d139" = 19.14
  dimension "d140" = 19.14
  dimension "d141" = 135
  dimension "d142" = 135
  dimension "d143" = 3.08
  dimension "d144" = 3.08
  dimension "d145" = 3.3
  dimension "d146" = 4.4
  dimension "d147" = 3.3
  dimension "d148" = 3.3
  dimension "d149" = 4.4
  dimension "d150" = 3.3
  dimension "d151" = 3.3
  dimension "d152" = 2.42
  dimension "d153" = 3.3
  dimension "d154" = 4.62
  dimension "d155" = 4.62
  dimension "d156" = 3.08
  dimension "d157" = 4.4
  dimension "d158" = 3.3
  dimension "d159" = 3.74
  dimension "d160" = 4.4
  dimension "d161" = 3.74
  dimension "d162" = 0
  dimension "d163" = 3.3
  dimension "d164" = 135
  dimension "d165" = 3.3
  dimension "d166" = 135
  dimension "d167" = 4.4
  dimension "d168" = 45
  dimension "d169" = 3.3
  dimension "d170" = 3.3
  dimension "d171" = 45
  dimension "d172" = 3.3
  dimension "d173" = 91.96
  dimension "d174" = 22.44
  dimension "d175" = 3.08
  constraints: 218 end point, 29 perpendicular, 18 point on line, 16 collinear, 11 horizontal, 8 midpoint, 6 parallel, 5 vertical, 4 horizontal alignment, 2 vertical alignment, 1 coincident, 1 equal length, 6 other
  measures "d137" distance of L37.end L45.start
  measures "d138" distance of L37.start L37.end
  measures "d139" distance of point (0, -121.52) point (-19.14, -121.52)
  measures "d140" distance of point (0, -121.52) point (19.14, -121.52)
  measures "d141" angle of L109 L53
  measures "d142" angle of L48 L51
  measures "d143" distance between parallel lines of L49 L37
  measures "d144" distance between parallel lines of L53 L51
  measures "d145" vertical distance of point (0, -121.52) L48.end
  measures "d146" distance from line of L60 L109.end
  measures "d147" distance of L62.start L91.start
  measures "d148" distance between parallel lines of L85 L87
  measures "d149" distance between parallel lines of L41 L86
  measures "d150" distance of L79.start L80.start
  measures "d151" distance between parallel lines of L81 L78
  measures "d152" distance of L80.start L80.end
  measures "d153" distance between parallel lines of L93 L84
  measures "d154" distance of L72.end L68.start
  measures "d155" distance of L71.end L66.end
  measures "d156" distance between parallel lines of L65 L64
  measures "d157" distance of L73.end L75.end
  measures "d158" distance between parallel lines of L70 L73
  measures "d159" distance between parallel lines of L11 L19
  measures "d160" distance between parallel lines of L15 L8
  measures "d161" distance between parallel lines of L16 L7
  measures "d162" distance of point (32.833, -110.3) L102.start
  measures "d163" distance between parallel lines of L22 L31
  measures "d164" angle of L24 L33
  measures "d165" distance between parallel lines of L29 L27
  measures "d166" angle of L35 L36
  measures "d167" distance between parallel lines of L21 L25
  measures "d168" angle of L96 L97
  measures "d169" distance between parallel lines of L98 L100
  measures "d170" distance between parallel lines of L20 L95
  measures "d171" angle of L99 L100
  measures "d172" distance of L97.end L18.end
  measures "d173" distance between parallel lines of L66 L22
  measures "d174" distance of L22.end L21.end
  measures "d175" distance between parallel lines of L45 L108
extrude "Extrusion13" cut sketch "Sketch13" against normal blind 0.1
equation "\"d0\" = wSupply"
equation "\"d1\" = lSupply"
equation "\"d4\" = lPanel"
equation "\"d5\" = wPanel"
equation "\"wSupply\" = 109"
equation "\"lSupply\" = 257.5"
equation "\"lPanel\" = 40.6"
equation "\"wPanel\" = 81.6"
body "Solid1"
